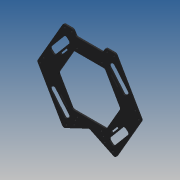
# Autodesk Inventor part: Bottom Plate
Saved by Autodesk Inventor 2017 (Build 210142000, 142)
## iProperties
Created: 2016-10-01
Part Number: Bottom Plate
Material: PVC, Unplasticized
Document SubType Name: Modeling
Designer: James Yelland
Density: 1.29 g/cm^3
Appearance: Smooth - White
Mass: 37.5584 g
Surface Area: 327.952 cm^2
Volume: 29.115 cm^3
Author: James Yelland
Autodesk Inventor part; units mm, degrees
ref_plane "YZ Plane" through (0, 0, 0) normal (1, 0, 0) x (0, 1, 0)
ref_plane "XZ Plane" through (0, 0, 0) normal (0, 1, 0) x (-1, 0, 0)
ref_plane "XY Plane" through (0, 0, 0) normal (0, 0, 1) x (1, 0, 0)
sketch "Sketch1" plane through (0, 0, 0) normal (0, 1, 0) x (-1, 0, 0)
  line L0 (103.5566, -2.5) -> (54.8095, -86.9325)
  line L1 (-54.8095, -86.9325) -> (-103.5566, -2.5)
  line L2 (-103.5566, 2.5) -> (-53.9434, 88.4327)
  line L3 (53.9434, 88.4327) -> (103.5566, 2.5)
  arc A0 (48.3297, -88.9468) -> (54.8095, -86.9325) centre (50.4794, -84.4325) ccw
  arc A1 (-54.8095, -86.9325) -> (-48.3297, -88.9468) centre (-50.4794, -84.4325) ccw
  arc A2 (-103.5566, 2.5) -> (-103.5566, -2.5) centre (-99.2265, 0) ccw
  arc A3 (-49.6132, 90.9327) -> (-53.9434, 88.4327) centre (-49.6132, 85.9327) ccw
  arc A4 (53.9434, 88.4327) -> (49.6132, 90.9327) centre (49.6132, 85.9327) ccw
  arc A5 (103.5566, -2.5) -> (103.5566, 2.5) centre (99.2265, 0) ccw
  circle A6 centre (49.6132, 85.9327) radius 1.6
  circle A7 centre (-49.6132, 85.9327) radius 1.6
  circle A8 centre (-99.2265, 0) radius 1.6
  circle A9 centre (99.2265, 0) radius 1.6
  circle A10 centre (-25, 62.282) radius 1.6
  circle A11 centre (25, 62.282) radius 1.6
  circle A12 centre (24, -57.282) radius 1.6
  circle A13 centre (-24, -57.282) radius 1.6
  circle A14 centre (-30.6147, -73.9104) radius 1.6
  circle A15 centre (30.6147, -73.9104) radius 1.6
  circle A16 centre (35.5991, 85.9437) radius 1.6
  circle A17 centre (-35.5945, 85.9327) radius 1.6
  circle A18 centre (92.2171, 12.1406) radius 1.6
  circle A19 centre (-92.2171, 12.1406) radius 1.6
  arc A20 (31.3397, -49.282) -> (35.6699, -46.782) centre (31.3397, -44.282) ccw
  line L4 (31.3397, -49.282) -> (-31.3397, -49.282)
  arc A21 (-35.6699, -46.782) -> (-31.3397, -49.282) centre (-31.3397, -44.282) ccw
  line L5 (-35.6699, -46.782) -> (-61.2361, -2.5)
  arc A22 (-61.2361, 2.5) -> (-61.2361, -2.5) centre (-56.906, 0) ccw
  line L6 (-61.2361, 2.5) -> (-32.7831, 51.782)
  arc A23 (-28.453, 54.282) -> (-32.7831, 51.782) centre (-28.453, 49.282) ccw
  line L7 (-28.453, 54.282) -> (28.453, 54.282)
  arc A24 (32.7831, 51.782) -> (28.453, 54.282) centre (28.453, 49.282) ccw
  line L8 (32.7831, 51.782) -> (61.2361, 2.5)
  arc A25 (61.2361, -2.5) -> (61.2361, 2.5) centre (56.906, 0) ccw
  line L9 (61.2361, -2.5) -> (35.6699, -46.782)
  arc A26 (67.8361, 29.5077) -> (73.4714, 29.0147) centre (70.9003, 32.0789) ccw
  arc A27 (77.3017, 32.2286) -> (77.7947, 37.8639) centre (74.7305, 35.2928) ccw
  line L10 (73.4714, 29.0147) -> (77.3017, 32.2286)
  arc A28 (50.7976, 70.0378) -> (45.1623, 70.5308) centre (47.7335, 67.4666) ccw
  line L11 (45.1623, 70.5308) -> (41.3321, 67.3169)
  arc A29 (41.3321, 67.3169) -> (40.8391, 61.6815) centre (43.9032, 64.2527) ccw
  line L12 (64.2962, 53.9509) -> (50.7976, 70.0378)
  line L13 (64.2962, 53.9509) -> (77.7947, 37.8639)
  line L14 (40.8391, 61.6815) -> (67.8361, 29.5077)
  line L15 (49.7796, 41.77) -> (43.3517, 49.4305)
  line L16 (43.3517, 49.4305) -> (45.6499, 51.3589)
  line L17 (45.6499, 51.3589) -> (58.5056, 36.038)
  line L18 (58.5056, 36.038) -> (56.2075, 34.1096)
  line L19 (56.2075, 34.1096) -> (49.7796, 41.77)
  arc A30 (73.4714, -29.0147) -> (67.8361, -29.5077) centre (70.9003, -32.0789) ccw
  line L20 (54.3376, -45.5946) -> (57.5515, -41.7644)
  line L21 (45.6499, -51.3589) -> (58.5056, -36.038)
  line L22 (58.5056, -36.038) -> (56.2075, -34.1096)
  line L23 (40.8391, -61.6815) -> (67.8361, -29.5077)
  line L24 (64.2962, -53.9509) -> (77.7947, -37.8639)
  line L25 (73.4714, -29.0147) -> (77.3017, -32.2286)
  arc A31 (77.7947, -37.8639) -> (77.3017, -32.2286) centre (74.7305, -35.2928) ccw
  line L26 (43.3517, -49.4305) -> (45.6499, -51.3589)
  line L27 (49.7796, -41.77) -> (43.3517, -49.4305)
  arc A32 (45.1623, -70.5308) -> (50.7976, -70.0378) centre (47.7335, -67.4666) ccw
  line L28 (64.2962, -53.9509) -> (50.7976, -70.0378)
  line L29 (45.1623, -70.5308) -> (41.3321, -67.3169)
  arc A33 (40.8391, -61.6815) -> (41.3321, -67.3169) centre (43.9032, -64.2527) ccw
  line L30 (56.2075, -34.1096) -> (49.7796, -41.77)
  line L31 (-40.8391, -61.6815) -> (-67.8361, -29.5077)
  arc A34 (-67.8361, -29.5077) -> (-73.4714, -29.0147) centre (-70.9003, -32.0789) ccw
  line L32 (-45.6499, -51.3589) -> (-58.5056, -36.038)
  line L33 (-64.2962, -53.9509) -> (-77.7947, -37.8639)
  line L34 (-73.4714, -29.0147) -> (-77.3017, -32.2286)
  arc A35 (-77.3017, -32.2286) -> (-77.7947, -37.8639) centre (-74.7305, -35.2928) ccw
  line L35 (-43.3517, -49.4305) -> (-45.6499, -51.3589)
  line L36 (-49.7796, -41.77) -> (-43.3517, -49.4305)
  line L37 (-56.2075, -34.1096) -> (-49.7796, -41.77)
  line L38 (-45.1622, -70.5309) -> (-41.332, -67.3169)
  arc A36 (-50.7976, -70.0378) -> (-45.1622, -70.5309) centre (-47.7334, -67.4668) ccw
  line L39 (-64.2962, -53.9509) -> (-50.7976, -70.0378)
  arc A37 (-41.332, -67.3169) -> (-40.8391, -61.6815) centre (-43.9032, -64.2528) ccw
  line L40 (-40.8391, 61.6815) -> (-67.8361, 29.5077)
  arc A38 (-73.4714, 29.0147) -> (-67.8361, 29.5077) centre (-70.9003, 32.0789) ccw
  line L41 (-73.4714, 29.0147) -> (-77.3017, 32.2286)
  arc A39 (-77.7947, 37.8639) -> (-77.3017, 32.2286) centre (-74.7305, 35.2928) ccw
  line L42 (-64.2962, 53.9509) -> (-77.7947, 37.8639)
  line L43 (-56.2075, 34.1096) -> (-49.7796, 41.77)
  line L44 (-49.7796, 41.77) -> (-43.3517, 49.4305)
  line L45 (-45.6499, 51.3589) -> (-58.5056, 36.038)
  line L46 (-58.5056, 36.038) -> (-56.2075, 34.1096)
  line L47 (-64.2962, 53.9509) -> (-50.7976, 70.0378)
  line L48 (-43.3517, 49.4305) -> (-45.6499, 51.3589)
  line L49 (-45.1623, 70.5308) -> (-41.3321, 67.3169)
  arc A40 (-45.1623, 70.5308) -> (-50.7976, 70.0378) centre (-47.7335, 67.4666) ccw
  arc A41 (-40.8391, 61.6815) -> (-41.3321, 67.3169) centre (-43.9032, 64.2527) ccw
  line L50 (-56.2075, -34.1096) -> (-58.5056, -36.038)
  circle A42 centre (28.2679, -64.7457) radius 1.6
  circle A43 centre (-28.2679, -64.7457) radius 1.6
  line L51 (48.2265, -83.602) -> (45.2265, -83.602)
  line L52 (45.2265, -83.602) -> (45.2265, -77.602)
  line L53 (45.2265, -77.602) -> (48.2265, -77.602)
  line L54 (48.2265, -77.602) -> (48.2265, -83.602)
  line L55 (-45.2265, -83.602) -> (-48.2265, -83.602)
  line L56 (-48.2265, -83.602) -> (-48.2265, -77.602)
  line L57 (-48.2265, -77.602) -> (-45.2265, -77.602)
  line L58 (-45.2265, -77.602) -> (-45.2265, -83.602)
  line L59 (0, 80.9327) -> (24.1132, 80.9327)
  line L60 (28.4434, 83.4327) -> (31.3301, 88.4327)
  line L61 (0, 80.9327) -> (-24.1132, 80.9327)
  line L62 (-28.4434, 83.4327) -> (-31.3301, 88.4327)
  line L63 (49.6132, 90.9327) -> (35.6603, 90.9327)
  line L64 (-35.6603, 90.9327) -> (-49.6132, 90.9327)
  arc A44 (35.6603, 90.9327) -> (31.3301, 88.4327) centre (35.6603, 85.9327) ccw
  arc A45 (-31.3301, 88.4327) -> (-35.6603, 90.9327) centre (-35.6603, 85.9327) ccw
  arc A46 (24.1132, 80.9327) -> (28.4434, 83.4327) centre (24.1132, 85.9327) ccw
  arc A47 (-28.4434, 83.4327) -> (-24.1132, 80.9327) centre (-24.1132, 85.9327) ccw
  line L65 (48.3297, -88.9468) -> (2.1402, -66.9602)
  line L66 (-2.1585, -66.9605) -> (-48.3297, -88.9468)
  arc A48 (2.1402, -66.9602) -> (-2.1585, -66.9605) centre (-0.0088, -71.4748) ccw
  point P0 (52.5, -90.9327)
  point P1 (-52.5, 90.9327)
  point P2 (52.5, 90.9327)
  point P3 (70.4073, 26.4435)
  point P4 (80.3658, 34.7998)
  point P5 (38.2679, 64.7457)
  point P6 (48.2265, 73.102)
  point P7 (54.3376, 45.5946)
  point P8 (57.5515, 41.7644)
  point P9 (70.4073, -26.4435)
  point P10 (80.3658, -34.7998)
  point P11 (-70.4073, -26.4435)
  point P12 (-83.093, -27.663)
  point P13 (-70.4073, 26.4435)
  point P14 (-80.3658, 34.7998)
  point P15 (-48.2265, 73.102)
  point P16 (-38.2679, 64.7457)
  point P17 (27, 80.9327)
  point P18 (-27, 80.9327)
  dimension "d11" = 360
  dimension "d30" = 360
  dimension "d90" = 360
  dimension "d136" = 360
  dimension "d180" = 3.2
  dimension "d181" = 6
  dimension "d182" = 6
  dimension "d184" = 27
  dimension "d185" = 120
  dimension "d186" = 27
  dimension "d187" = 120
  dimension "d188" = 5
  dimension "d189" = 5
  dimension "d200" = 5
  constraints: 134 end point, 66 point on circle, 55 centre point, 31 point on line, 10 tangent, 6 coincident, 5 equal length, 2 equal radius, 2 horizontal, 2 perpendicular, 1 midpoint
  measures "d180" diameter of A43
  measures "d181" distance of L51.end L52.end
  measures "d182" distance of L55.end L56.end
  measures "d184" distance of L59.start point (27, 80.933)
  measures "d185" angle of L60 L59
  measures "d186" distance of L59.start point (-27, 80.933)
  measures "d187" angle of L61 L62
  measures "d188" radius of A44
  measures "d189" radius of A46
  measures "d200" radius of A48
extrude "Extrusion1" add sketch "Sketch1" along normal blind 3
body "Solid1"
